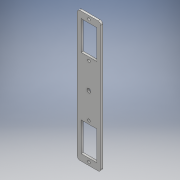
# Autodesk Inventor part: ramie2
Saved by Autodesk Inventor 2017.3 (Build 213256000, 256)
## iProperties
Created: 2019-03-17
Part Number: ramie2
Material: Ogólny
Document SubType Name: Modeling
Designer: legox
Density: 1 g/cm^3
Appearance: Domyślna
Author: legox
Autodesk Inventor part; units mm, degrees
ref_plane "YZ Plane" through (0, 0, 0) normal (1, 0, 0) x (0, 1, 0)
ref_plane "XZ Plane" through (0, 0, 0) normal (0, 1, 0) x (-1, 0, 0)
ref_plane "XY Plane" through (0, 0, 0) normal (0, 0, 1) x (1, 0, 0)
sketch "Szkic1" plane through (0, 0, 0) normal (0, 1, 0) x (-1, 0, 0)
  line L0 (-2, 0) -> (-16, 0)
  line L1 (-18, -2) -> (-18, -98)
  line L2 (-16, -100) -> (-2, -100)
  line L3 (0, -98) -> (0, -2)
  line L4 (-3, -5) -> (-15, -5)
  line L5 (-15, -5) -> (-15, -27.5)
  line L6 (-15, -27.5) -> (-3, -27.5)
  line L7 (-3, -27.5) -> (-3, -5)
  circle A0 centre (-9, -2.4) radius 1
  circle A1 centre (-9, -30.1) radius 1
  circle A2 centre (-9, -50) radius 1.5
  line L8 (-3, -95) -> (-15, -95)
  line L9 (-15, -95) -> (-15, -72.5)
  line L10 (-15, -72.5) -> (-3, -72.5)
  line L11 (-3, -72.5) -> (-3, -95)
  circle A3 centre (-9, -97.6) radius 1
  circle A4 centre (-9, -69.9) radius 1
  arc A5 (0, -2) -> (-2, 0) centre (-2, -2) ccw
  arc A6 (-16, 0) -> (-18, -2) centre (-16, -2) ccw
  arc A7 (-18, -98) -> (-16, -100) centre (-16, -98) ccw
  arc A8 (-2, -100) -> (0, -98) centre (-2, -98) ccw
  point P0 (0, 0)
  point P1 (-18, -100)
  point P2 (-18, 0)
  point P3 (0, -100)
  dimension "d0" = 18
  dimension "d1" = 100
  dimension "d2" = 12
  dimension "d3" = 22.5
  dimension "d4" = 2
  dimension "d5" = 2.6
  dimension "d6" = 6
  dimension "d7" = 5
  dimension "d8" = 2
  dimension "d9" = 2.6
  dimension "d10" = 6
  dimension "d11" = 3
  dimension "d12" = 2
  constraints: 24 end point, 9 centre point, 8 point on circle, 8 point on line, 8 tangent, 4 parallel, 3 equal radius, 2 horizontal, 2 perpendicular
  measures "d0" distance of point (0, -100) point (-18, -100)
  measures "d1" distance of point (-18, -100) point (-18, 0)
  measures "d2" distance of L6.end L5.end
  measures "d3" distance of L5.end L4.end
  measures "d4" diameter of A0
  measures "d5" distance from line of L4 A0.centre
  measures "d6" distance from line of L5 A0.centre
  measures "d7" distance between parallel lines of L0 L4
  measures "d8" diameter of A1
  measures "d9" distance from line of L6 A1.centre
  measures "d10" distance from line of L5 A1.centre
  measures "d11" diameter of A2
  measures "d12" radius of A5
extrude "Wyciągnięcie proste1" add sketch "Szkic1" along normal blind 1.6
equation "\"d6\" = 0.5 * d2"
equation "\"d10\" = 0.5 * d2"
